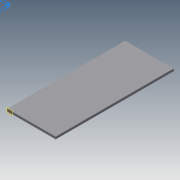
# Autodesk Inventor part: Z-table
Saved by Autodesk Inventor 2014 SP1 (Build 180222100, 222)
## iProperties
Created: 2014-04-10
Part Number: Z-table
Material: Generic
Document SubType Name: Modeling
Designer: tom
Density: 1 g/cm^3
Appearance: Default
Author: tom
Autodesk Inventor part; units mm, degrees
ref_plane "YZ Plane" through (0, 0, 0) normal (1, 0, 0) x (0, 1, 0)
ref_plane "XZ Plane" through (0, 0, 0) normal (0, 1, 0) x (-1, 0, 0)
ref_plane "XY Plane" through (0, 0, 0) normal (0, 0, 1) x (1, 0, 0)
ref_plane "Work Plane1" through (33.3916, -139.4155, 142.8527) normal (0, 0, 1) x (1, 0, 0)
sketch "Sketch1" plane through (33.3916, -139.4155, 142.8527) normal (0, 0, 1) x (1, 0, 0)
  line L0 (-4.0384, 3.4) -> (113.4116, 3.4)
  line L1 (54.6866, 21.1837) -> (54.6866, -18.7057) construction
  line L2 (-4.0384, 3.4) -> (-4.0384, -2.26)
  line L3 (-4.0384, -2.26) -> (113.4116, -2.26)
  line L4 (113.4116, -2.26) -> (113.4116, 3.4)
  dimension "d0" = 5.66
  constraints: 10 end point, 3 perpendicular, 1 parallel
  measures "d0" distance of L0.start L2.end
extrude "Extrusion1" add sketch "Sketch1" against normal blind 286.324
body "Solid1"
